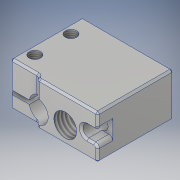
# Autodesk Inventor part: E3D-v6 Volcano Heater Block
Saved by Autodesk Inventor 2018.2 (Build 222227000, 227)
## iProperties
Created: 2018-02-27
Part Number: E3D-v6 Volcano Heater Block
Material: Aluminium 6061
Document SubType Name: Modeling
Designer: Till
Density: 2.7 g/cm^3
Appearance: Aluminium - flach
Author: Till
Autodesk Inventor part; units mm, degrees
ref_plane "YZ Plane" through (0, 0, 0) normal (1, 0, 0) x (0, 1, 0)
ref_plane "XZ Plane" through (0, 0, 0) normal (0, 1, 0) x (-1, 0, 0)
ref_plane "XY Plane" through (0, 0, 0) normal (0, 0, 1) x (1, 0, 0)
sketch "Skizze1" plane through (0, 0, 0) normal (0, 0, 1) x (1, 0, 0)
  line L0 (0, 0) -> (0, -20)
  line L1 (0, -20) -> (-16, -20)
  line L2 (-16, -20) -> (-16, -19)
  line L3 (-16, -19) -> (-24, -19)
  line L4 (-24, -19) -> (-24, 0)
  line L5 (-24, 0) -> (0, 0)
  dimension "d0" = 20
  dimension "d1" = 16
  dimension "d2" = 1
  dimension "d3" = 8
  constraints: 12 end point, 5 perpendicular, 1 vertical
  measures "d0" distance of L0.start L0.end
  measures "d1" distance of L0.end L1.end
  measures "d2" distance of L1.end L2.end
  measures "d3" distance of L2.end L3.end
extrude "Main Body" add sketch "Skizze1" along normal blind 11.5
sketch "Skizze2" plane through (-24, 0, 0) normal (0, 1, 0) x (1, 0, 0)
  arc A0 (5.042, -4.5) -> (5.042, -3.5) centre (8, -4) ccw
  line L0 (0, 0) -> (0, -11.5) projected
  line L1 (24, -11.5) -> (0, -11.5) projected
  line L2 (5.042, -3.5) -> (0, -3.5)
  line L3 (5.042, -4.5) -> (0, -4.5)
  line L4 (0, -3.5) -> (0, -4.5)
  circle A1 centre (15.5, -4.5) radius 3
  circle A2 centre (21.2, -5.75) radius 1.55
  line L5 (0, 0) -> (24, 0) projected
  dimension "d6" = 8
  dimension "d7" = 3
  dimension "d9" = 1
  dimension "d10" = 0.5
  dimension "d11" = 6
  dimension "d13" = 15.5
  dimension "d14" = 3.1
  dimension "d15" = 21.2
  dimension "d19" = 4
  dimension "d20" = 4.5
  dimension "d21" = 5.75
  constraints: 6 end point, 3 centre point, 2 perpendicular, 2 point on circle, 2 point on line, 1 collinear
  measures "d6" distance from line of L0 A0.centre
  measures "d7" radius of A0
  measures "d9" distance between parallel lines of L3 L2
  measures "d10" distance from line of A0.centre L3
  measures "d11" diameter of A1
  measures "d13" distance from line of L0 A1.centre
  measures "d14" diameter of A2
  measures "d15" distance from line of L0 A2.centre
  measures "d19" distance from line of L5 A0.centre
  measures "d20" distance from line of L5 A1.centre
  measures "d21" distance from line of L5 A2.centre
extrude "Insert Holes" cut sketch "Skizze2" against normal through all
sketch "Skizze3" plane through (-16, -20, 0) normal (0, -1, 0) x (1, 0, 0)
  circle A0 centre (13.2, 5.75) radius 1.55 projected
  line L0 (13.2, 7.3) -> (16, 7.3)
  line L1 (13.2, 4.2) -> (16, 4.2)
  line L2 (16, 0) -> (16, 11.5) projected
  line L3 (16, 4.2) -> (16, 7.3)
  line L4 (13.2, 7.3) -> (13.2, 4.2)
  constraints: 8 end point, 2 horizontal, 2 point on circle, 1 parallel, 1 perpendicular, 1 point on line, 1 tangent
extrude "Cable Opening" cut sketch "Skizze3" against normal blind 4 contours A0 L0 L2 L1
fillet "Rundung1" radius 1 6 edges at (-16, -19, 9.25) (-16, -19, 0.5) (0, -18, 7.3) (0, -18, 4.2) (-16, -20, 9.25) (-16, -20, 0.5)
sketch "Skizze4" plane through (0, 0, 0) normal (0, 0, -1) x (-1, 0, 0)
  circle A0 centre (21.5, -15) radius 1.5
  circle A1 centre (21.5, -5.5) radius 1.5
  line L0 (24, -19) -> (24, 0) projected
  line L1 (24, 0) -> (0, 0) projected
  dimension "d25" = 3
  dimension "d26" = 3
  dimension "d27" = 2.5
  dimension "d28" = 2.5
  dimension "d29" = 5.5
  dimension "d30" = 15
  constraints: 2 centre point
  measures "d25" diameter of A0
  measures "d26" diameter of A1
  measures "d27" distance from line of L0 A0.centre
  measures "d28" distance from line of L0 A1.centre
  measures "d29" distance from line of L1 A1.centre
  measures "d30" distance from line of L1 A0.centre
extrude "Cartridge clamping holes" cut sketch "Skizze4" against normal through all
sketch "Skizze5" plane through (0, 0, 0) normal (0, 0, -1) x (-1, 0, 0)
  circle A0 centre (2.8, -10) radius 1.5
  line L0 (24, -19) -> (24, 0) projected
  line L1 (24, 0) -> (0, 0) projected
  dimension "d33" = 3
  dimension "d34" = 21.2
  dimension "d35" = 10
  constraints: 1 centre point
  measures "d33" diameter of A0
  measures "d34" distance from line of L0 A0.centre
  measures "d35" distance from line of L1 A0.centre
extrude "PT100 clamping holes" cut sketch "Skizze5" against normal up to next
chamfer "Fase1" distance 0.5 angle 45 24 edges at (0, -10, 11.5) (-7.6338, -20, 11.5) (-15.7677, -19.866, 11.5) (-20.4995, -19, 11.5) (-7.6338, -20, 0) (-15.7677, -19.866, 0) (-20.4995, -19, 0) (0, -10, 0) (0, 0, 5.75) (-12, 0, 11.5) (-24, -19, 8) (-24, -9.5, 11.5) (-24, -19, 1.75) (0, -20, 9.9) (-0.2929, -20, 7.5929) (-1.9, -20, 7.3) (-4.35, -20, 5.75) (-1.9, -20, 4.2) (-0.2929, -20, 3.9071) (0, -20, 1.6) (-12, 0, 0) (-24, -9.5, 0) (-24, 0, 1.75) (-24, 0, 8)
thread "Gewinde1" size "M6x1" class "6H" standard "ANSI Metric M Profile" full length
thread "Gewinde2" size "M3x0.5" class "6H" standard "ANSI Metric M Profile" full length
thread "Gewinde3" size "M3x0.5" class "6H" standard "ANSI Metric M Profile" full length
thread "Gewinde4" size "M3x0.5" class "6H" standard "ANSI Metric M Profile" full length
